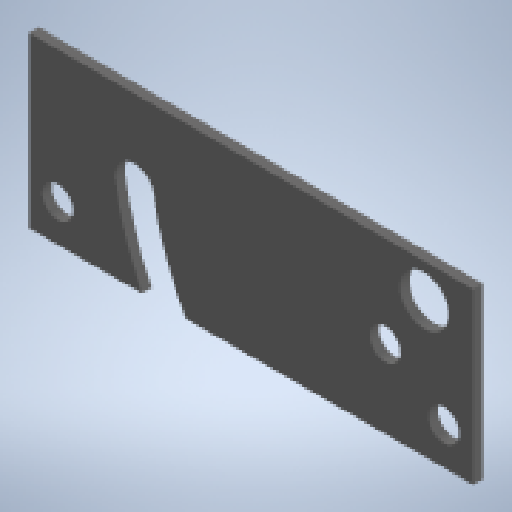
# Autodesk Inventor part: battery_holder_cover
Saved by Autodesk Inventor 2024.1 (Build 281209000, 209)
## iProperties
Created: 2025-03-30
Part Number: battery_holder_cover
Material: 一般
Document SubType Name: Modeling
Designer: hibik
Density: 1 g/cm^3
Appearance: 既定
Author: hibik
Autodesk Inventor part; units mm, degrees
ref_plane "YZ Plane" through (0, 0, 0) normal (1, 0, 0) x (0, 1, 0)
ref_plane "XZ Plane" through (0, 0, 0) normal (0, 1, 0) x (-1, 0, 0)
ref_plane "XY Plane" through (0, 0, 0) normal (0, 0, 1) x (1, 0, 0)
sketch "スケッチ1" plane through (0, 0, 0) normal (0, 0, 1) x (1, 0, 0)
  line L0 (0, 0) -> (45.4, 0)
  line L1 (45.4, 0) -> (45.4, 17.3)
  line L2 (45.4, 17.3) -> (0, 17.3)
  line L3 (0, 17.3) -> (0, 0)
  dimension "d0" = 45.4
  dimension "d1" = 17.3
  constraints: 8 end point, 2 parallel, 1 horizontal, 1 perpendicular
  measures "d0" distance of L2.end L1.end
  measures "d1" distance of L1.end L0.end
extrude "押し出し1" add sketch "スケッチ1" along normal blind 1
sketch "スケッチ2" plane through (0, 0, 0) normal (0, 0, -1) x (-1, 0, 0)
  circle A0 centre (-40.4, 13.8) radius 2.25 projected
  circle A1 centre (-36.4, 7.9571) radius 1.35 projected
  circle A2 centre (-42.4, 3.8) radius 1.35 projected
  circle A3 centre (-2.9, 3.8) radius 1.35 projected
  arc A4 (-14.4192, -1.2) -> (-10.4845, 16.05) centre (-40.4, 13.8) ccw
  line L0 (-40.4, 16.05) -> (-10.4845, 16.05)
  line L1 (-40.4, 13.8) -> (-14.4192, -1.2)
  circle A5 centre (-14.4192, -1.2) radius 2
  arc A6 (-16.1513, -0.2) -> (-12.4905, 16.05) centre (-40.4, 13.8) ccw
  arc A7 (-12.6872, -2.2) -> (-8.4011, 14.0667) centre (-40.4, 13.8) ccw
  circle A8 centre (-36.4, 7.9571) radius 1.6
  circle A9 centre (-42.4, 3.8) radius 1.6
  circle A10 centre (-40.4, 13.8) radius 2.5
  circle A11 centre (-2.9, 3.8) radius 1.6
  circle A12 centre (-10.7693, 9.107) radius 2
  line L2 (-40.4, 13.8) -> (-10.7693, 9.107)
  point P0 (0, 0)
  point P1 (-12.7447, 9.4198)
  point P2 (-8.794, 8.7941)
  point P3 (-11.1479, 7.1431)
  point P4 (-10.5225, 11.0917)
  dimension "d4" = 30
  dimension "d5" = 30
  dimension "d6" = 4
  dimension "d7" = 3.2
  dimension "d8" = 3.2
  dimension "d9" = 5
  dimension "d10" = 3.2
  dimension "d13" = 9
  constraints: 10 point on circle, 9 centre point, 6 coincident, 6 end point, 3 concentric, 2 horizontal, 2 point on line, 2 tangent, 1 vertical alignment, 1 other
  measures "d4" radius of A4
  measures "d5" angle of L0 L1
  measures "d6" diameter of A5
  measures "d7" diameter of A8
  measures "d8" diameter of A9
  measures "d9" diameter of A10
  measures "d10" diameter of A11
  measures "d13" angle of L0 L2
extrude "押し出し2" cut sketch "スケッチ2" against normal through all contours A0 L2 L1 | A0 L0 A10 L2 | A0 L1 A10 L0 | L2 A10 L1 A0 | A0 L1 L2 | A12 A4 A5 A6 | L2 A4 A12 | A12 A4 L2 | A5 A4 L1 | L1 A4 A5 | A12 A4 | A12 A7 A5 A4 | A1 | A2 | A3 | A8 | A9 | A11
